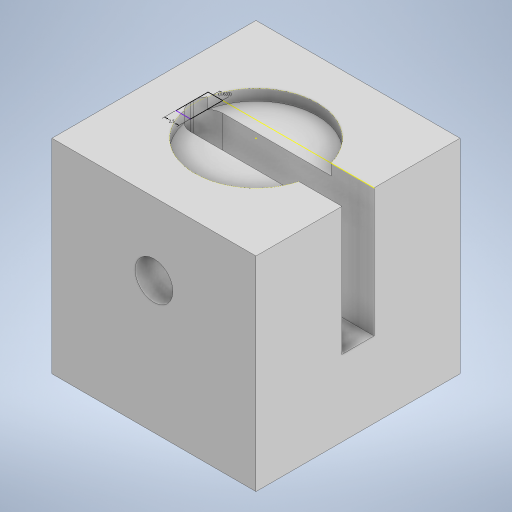
# Autodesk Inventor part: Holder
Saved by Autodesk Inventor 2024 (Build 280153000, 153)
## iProperties
Created: 2026-03-08
Part Number: Holder
Material: Generic
Document SubType Name: Modeling
Designer: Nathan
Density: 1 g/cm^3
Appearance: Default
Author: Nathan
Autodesk Inventor part; units mm, degrees
ref_plane "YZ Plane" through (0, 0, 0) normal (1, 0, 0) x (0, 1, 0)
ref_plane "XZ Plane" through (0, 0, 0) normal (0, 1, 0) x (-1, 0, 0)
ref_plane "XY Plane" through (0, 0, 0) normal (0, 0, 1) x (1, 0, 0)
sketch "Sketch1" plane through (0, 0, 0) normal (0, 1, 0) x (-1, 0, 0)
  line L0 (17.5, 17.5) -> (-17.5, 17.5)
  line L1 (-17.5, 17.5) -> (-17.5, -17.5)
  line L2 (-17.5, -17.5) -> (17.5, -17.5)
  line L3 (17.5, -17.5) -> (17.5, 17.5)
  line L4 (17.5, 17.5) -> (-17.5, -17.5) construction
  line L5 (-17.5, 17.5) -> (17.5, -17.5) construction
  point P0 (0, 0)
  dimension "d0" = 35
  dimension "d1" = 35
  constraints: 12 end point, 2 midpoint, 2 parallel, 1 horizontal, 1 perpendicular
  measures "d0" distance of L2.end L1.end
  measures "d1" distance of L1.end L0.end
extrude "Extrusion1" add sketch "Sketch1" along normal blind 35
sketch "Sketch2" plane through (0, 35, 0) normal (0, 1, 0) x (1, 0, 0)
  line L0 (-2.3616, -50.7705) -> (15.6384, -50.7705)
  line L1 (15.6384, -50.7705) -> (15.6384, -44.7705)
  line L2 (15.6384, -44.7705) -> (-2.3616, -44.7705)
  line L3 (-2.3616, -44.7705) -> (-2.3616, -50.7705)
  line L4 (-2.3616, -50.7705) -> (15.6384, -44.7705) construction
  line L5 (15.6384, -50.7705) -> (-2.3616, -44.7705) construction
  circle A0 centre (6.6384, -47.7705) radius 11
  line L6 (-10.8616, -65.2705) -> (24.1384, -65.2705)
  line L7 (24.1384, -65.2705) -> (24.1384, -30.2705)
  line L8 (24.1384, -30.2705) -> (-10.8616, -30.2705)
  line L9 (-10.8616, -30.2705) -> (-10.8616, -65.2705)
  line L10 (-10.8616, -65.2705) -> (24.1384, -30.2705) construction
  line L11 (24.1384, -65.2705) -> (-10.8616, -30.2705) construction
  circle A1 centre (6.6384, -47.7705) radius 28.5
  circle A2 centre (0, 0) radius 10.5
  line L12 (-8.5, 2.75) -> (8.5, 2.75)
  line L13 (8.5, 2.75) -> (8.5, -2.75)
  line L14 (8.5, -2.75) -> (-8.5, -2.75)
  line L15 (-8.5, -2.75) -> (-8.5, 2.75)
  line L16 (-8.5, 2.75) -> (8.5, -2.75) construction
  line L17 (8.5, 2.75) -> (-8.5, -2.75) construction
  point P0 (-38.3616, 79.7295)
  dimension "d4" = 18
  dimension "d5" = 6
  dimension "d6" = 22
  dimension "d7" = 35
  dimension "d8" = 35
  dimension "d9" = 21
  dimension "d10" = 17
  dimension "d11" = 5.5
  constraints: 36 end point, 6 midpoint, 6 parallel, 3 centre point, 3 coincident, 3 horizontal, 3 perpendicular
  measures "d4" distance of L2.end L1.end
  measures "d5" distance of L1.end L0.end
  measures "d6" diameter of A0
  measures "d7" distance of L8.end L7.end
  measures "d8" distance of L7.end L6.end
  measures "d9" diameter of A2
  measures "d10" distance of L13.end L14.end
  measures "d11" distance of L12.end L13.end
extrude "Extrusion2" cut sketch "Sketch2" against normal blind 22 contours L12 L13 L14 L15
extrude "Extrusion3" cut sketch "Sketch2" against normal blind 1.9 contours A2
sketch "Sketch3" plane through (-17.5, 0, 17.5) normal (0, 0, 1) x (1, 0, 0)
  line L0 (7, 35) -> (28, 35) construction
  line L1 (17.5, 35) -> (17.5, 22.6) construction
  point P0 (17.5, 0)
  dimension "d16" = 12.4
  constraints: 2 end point, 1 midpoint, 1 vertical
  measures "d16" distance of L1.start L1.end
hole "Hole1" at (0, 22.6, 17.5) direction (0, 0, -1) diameter 6.5 end through all clearance for "Hex Head Cap Screw ISO 24017" size "M6" standard "ISO"
sketch "Sketch4" plane through (0, 0, 0) normal (0, -1, 0) x (1, 0, 0)
  point P0 (0, 0)
hole "Hole2" at (0, 0, 0) direction (0, 1, 0) diameter 4.917 depth 11 thread size "M6x1" class "6H" standard "ANSI Metric M Profile"
sketch "Sketch6" plane through (0, 0, 0) normal (0, -1, 0) x (1, 0, 0)
  line L0 (-17.5, -17.5) -> (-17.5, 17.5) construction
  line L1 (17.5, 17.5) -> (-17.5, 17.5) construction
  line L2 (-17.5, 17.5) -> (-17.5, -17.5) construction
  line L3 (-17.5, -17.5) -> (17.5, -17.5) construction
  line L4 (17.5, -17.5) -> (17.5, 17.5) construction
  line L5 (17.5, 17.5) -> (-17.5, -17.5) construction
  line L6 (-17.5, 17.5) -> (17.5, -17.5) construction
  line L7 (9, -9) -> (-9, -9) construction
  line L8 (-9, -9) -> (-9, 9) construction
  line L9 (-9, 9) -> (9, 9) construction
  line L10 (9, 9) -> (9, -9) construction
  line L11 (9, -9) -> (-9, 9) construction
  line L12 (-9, -9) -> (9, 9) construction
  point P0 (0, 0)
  dimension "d63" = 18
  dimension "d64" = 18
  constraints: 24 end point, 4 midpoint, 4 parallel, 2 horizontal, 2 perpendicular, 1 point on line
  measures "d63" distance of L7.end L8.end
  measures "d64" distance of L8.end L9.end
hole "Hole3" at (9, 0, 9) at (-9, 0, -9) direction (0, 1, 0) diameter 5 depth 11
sketch "Sketch7" plane through (0, 35, 0) normal (0, 1, 0) x (1, 0, 0)
  line L0 (-8.5, 2.75) -> (8.5, 2.75) construction
  line L1 (8.5, 2.75) -> (17.5, 2.75) construction
  line L2 (17.5, -17.5) -> (17.5, 17.5) construction
  line L3 (8.5, 2.75) -> (8.5, -2.75) projected
  line L4 (17.5, 2.75) -> (8.5, 2.75)
  line L5 (8.5, 2.75) -> (8.5, -2.75)
  line L6 (8.5, -2.75) -> (17.5, -2.75)
  line L7 (17.5, -2.75) -> (17.5, 2.75)
  point P0 (0, 0)
  constraints: 10 end point, 2 horizontal, 2 parallel, 1 perpendicular, 1 point on line
extrude "Extrusion4" cut sketch "Sketch7" against normal up to surface (22 mm away)
sketch "Sketch8" plane through (0, 35, 0) normal (0, 1, 0) x (1, 0, 0)
  line L0 (17.5, 2.75) -> (-8.5, 2.75) projected
  line L1 (-8.5, 2.75) -> (-11, 2.75)
  line L2 (-11, 2.75) -> (-11, -2.75)
  line L3 (-11, -2.75) -> (-8.5, -2.75)
  line L4 (-8.5, -2.75) -> (-8.5, 2.75)
  line L5 (-8.5, 2.75) -> (-10.1335, 2.75) construction
  arc A0 (10.1335, 2.75) -> (10.1335, -2.75) centre (0, 0) ccw construction
  dimension "d44" = 2.5
  dimension "d45" = 1.6335
  constraints: 10 end point, 2 parallel, 1 horizontal, 1 perpendicular, 1 point on circle, 1 point on line
  measures "d44" distance of L3.end L2.end
  measures "d45" distance of L5.end L0.end
extrude "Extrusion5" cut sketch "Sketch8" against normal up to surface (22 mm away)
fillet "Fillet2" radius 2.5 2 edges at (-11, 24, 2.75) (-11, 24, -2.75)
body "Solid1"
